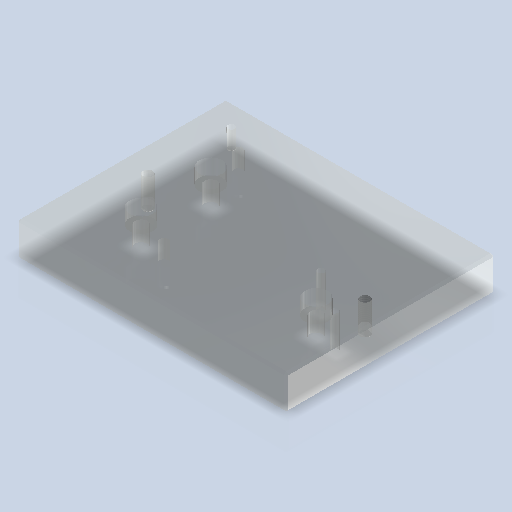
# Autodesk Inventor part: Grundplatte
Saved by Autodesk Inventor 2024.2 (Build 282272000, 272)
## iProperties
Created: 2024-04-22
Part Number: Grundplatte
Material: Glas
Document SubType Name: Modeling
Designer: Fabri
Density: 2.18 g/cm^3
Appearance: Klar
Author: Fabri
Autodesk Inventor part; units mm, degrees
note: some values were not read from the file. Chosen so that the rebuilt part matches the saved one: direction of "Bohrung5".
ref_plane "YZ Plane" through (0, 0, 0) normal (1, 0, 0) x (0, 1, 0)
ref_plane "XZ Plane" through (0, 0, 0) normal (0, 1, 0) x (-1, 0, 0)
ref_plane "XY Plane" through (0, 0, 0) normal (0, 0, 1) x (1, 0, 0)
sketch "Skizze1" plane through (0, 0, 0) normal (0, 0, 1) x (1, 0, 0)
  line L0 (-58, -45) -> (58, -45)
  line L1 (58, -45) -> (58, 45)
  line L2 (58, 45) -> (-58, 45)
  line L3 (-58, 45) -> (-58, -45)
  line L4 (-58, -45) -> (58, 45) construction
  line L5 (58, -45) -> (-58, 45) construction
  point P0 (0, 0)
  dimension "d0" = 116
  dimension "d1" = 90
  constraints: 12 end point, 2 midpoint, 2 parallel, 1 horizontal, 1 perpendicular
  measures "d0" distance between parallel lines of L1 L3
  measures "d1" distance between parallel lines of L0 L2
extrude "Extrusion1" add sketch "Skizze1" along normal blind 15
sketch "Skizze2" plane through (0, 0, 15) normal (0, 0, 1) x (1, 0, 0)
  line L0 (58, -45) -> (58, 45) projected
  point P0 (0, 0)
  point P1 (47, 0)
  point P2 (58, 0)
  dimension "d11" = 11
  constraints: 1 horizontal alignment, 1 midpoint
  measures "d11" distance from line of L0 point (47, 0)
hole "Bohrung1" at (47, 0, 15) direction (0, 0, -1) diameter 4.134 depth 13 tip angle 118 thread size "M5x0.8" class "6H" standard "ISO Metric profile"
sketch "Skizze4" plane through (0, 0, 15) normal (0, 0, 1) x (1, 0, 0)
  line L0 (-58, -45) -> (58, -45) projected
  line L1 (58, -45) -> (58, 45) projected
  point P0 (0, 0)
  point P1 (-35.5, 16)
  point P2 (36, -10)
  dimension "d20" = 35
  dimension "d21" = 61
  dimension "d22" = 22
  dimension "d23" = 71.5
  measures "d20" distance from line of L0 point (36, -10)
  measures "d21" distance from line of L0 point (-35.5, 16)
  measures "d22" distance from line of L1 point (36, -10)
  measures "d23" horizontal distance of point (-35.5, 16) point (36, -10)
hole "Bohrung3" at (-35.5, 16, 15) at (36, -10, 15) direction (0, 0, -1) diameter 5.5 end through all counterbore diameter 10 counterbore depth 6.5
sketch "Skizze5" plane through (0, 0, 15) normal (0, 0, 1) x (1, 0, 0)
  line L0 (-58, 45) -> (-58, -45) projected
  circle A0 centre (47, 0) radius 2.067 projected
  point P0 (0, 0)
  point P1 (-46.5721, 0)
  point P2 (-58, 0)
  dimension "d38" = 93.5721
  constraints: 1 horizontal alignment, 1 midpoint
  measures "d38" distance of A0.centre point (-46.572, 0)
hole "Bohrung4" at (-46.5721, 0, 15) direction (0, 0, -1) diameter 4.134 depth 13 tip angle 118 thread size "M5x0.8" class "6H" standard "ISO Metric profile"
sketch "Skizze6" plane through (0, 0, 15) normal (0, 0, 1) x (1, 0, 0)
  circle A0 centre (-35.5, 16) radius 2.75 projected
  point P0 (0, 0)
  point P1 (-35.5, -14)
  dimension "d39" = 30
  constraints: 1 vertical alignment
  measures "d39" distance of point (-35.5, -14) A0.centre
hole "Bohrung5" at (-35.5, -14, 15) direction (0, 0, -1) diameter 5.5 depth 15 counterbore diameter 10 counterbore depth 6.5
sketch "Skizze7" plane through (0, 0, 15) normal (0, 0, 1) x (1, 0, 0)
  point P0 (0, 0)
  point P1 (-46.0168, 35.3976)
hole "Bohrung6" at (-46.0168, 35.3976, 15) direction (0, 0, -1) diameter 3 depth 8 tip angle 118
sketch "Skizze8" plane through (0, 0, 0) normal (0, 0, -1) x (-1, 0, 0)
  line L0 (58, -45) -> (-58, -45) projected
  line L1 (58, 45) -> (58, -45) projected
  point P0 (0, 0)
  point P1 (42.6552, 35)
  point P2 (24.6552, -15)
  point P3 (58, 0)
  dimension "d61" = 50
  dimension "d62" = 30
  dimension "d63" = 18
  constraints: 1 midpoint
  measures "d61" vertical distance of point (24.655, -15) point (42.655, 35)
  measures "d62" distance from line of L0 point (24.655, -15)
  measures "d63" horizontal distance of point (42.655, 35) point (24.655, -15)
hole "Bohrung7" at (-42.6552, 35, 0) at (-24.6552, -15, 0) direction (0, 0, 1) diameter 4 depth 8 tip angle 118
sketch "Skizze10" plane through (0, 0, 0) normal (0, 0, -1) x (-1, 0, 0)
  line L0 (-58, -45) -> (-58, 45) projected
  line L1 (58, -45) -> (-58, -45) projected
  point P0 (0, 0)
  point P1 (-27, 1)
  point P2 (-45, -11)
  dimension "d71" = 18
  dimension "d72" = 31
  dimension "d73" = 34
  dimension "d74" = 12
  measures "d71" horizontal distance of point (-27, 1) point (-45, -11)
  measures "d72" distance from line of L0 point (-27, 1)
  measures "d73" distance from line of L1 point (-45, -11)
  measures "d74" vertical distance of point (-45, -11) point (-27, 1)
hole "Bohrung8" at (27, 1, 0) at (45, -11, 0) direction (0, 0, 1) diameter 3 end through all
chamfer "Fasen1" distance 1 angle 45 12 edges at (58, 0, 0) (0, 45, 0) (-58, 0, 0) (0, -45, 0) (0, 45, 15) (-58, 45, 7.5) (58, 45, 7.5) (-58, 0, 15) (58, 0, 15) (-58, -45, 7.5) (58, -45, 7.5) (0, -45, 15)
